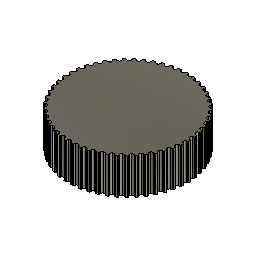
gear_53z (Autodesk Fusion 360 design; units mm, degrees)
Autodesk Fusion 360 part; units mm, degrees
sketch "Sketch1" plane through (0, 0, 0) normal (0, 0, 1) x (1, 0, 0) in component "gt2 pulley"
  circle A0 centre (0, 0) radius 16.8704 construction
  circle A1 centre (0, 0) radius 15.8664 construction
  line L0 (0, 0) -> (0, 16.8704) construction
  line L1 (0, 0) -> (0.9994, 16.8408) construction
  line L2 (0, 0) -> (1.4069, 16.8117) construction
  circle A2 centre (0, 0) radius 16.6164 construction
  arc A3 (0.389, 16.4769) -> (0.4579, 16.1856) centre (1.3857, 16.5585) ccw
  circle A4 centre (0, 0) radius 16.4664 construction
  arc A5 (0.2417, 16.6147) -> (0, 16.6164) centre (0, 0) ccw
  arc A6 (0.389, 16.4769) -> (0.2417, 16.6147) centre (0.2395, 16.4647) ccw
  arc A7 (0.4579, 16.1856) -> (0.9399, 15.8386) centre (0.9728, 16.3926) ccw
  arc A8 (0, 16.6164) -> (-0.2417, 16.6147) centre (0, 0) ccw
  arc A9 (-0.2417, 16.6147) -> (-0.389, 16.4769) centre (-0.2395, 16.4647) ccw
  arc A10 (-0.4579, 16.1856) -> (-0.389, 16.4769) centre (-1.3857, 16.5585) ccw
  arc A11 (-0.9399, 15.8386) -> (-0.4579, 16.1856) centre (-0.9728, 16.3926) ccw
  arc A12 (0.9399, 15.8386) -> (-0.9399, 15.8386) centre (0, 0) ccw
  point P0 (1.3857, 16.5585)
  point P1 (0, 16.6164)
  dimension "d18" = 33.7408
  dimension "d19" = 3.396
  dimension "d22" = 1.004
  dimension "d24" = 0.75
  dimension "d26" = 1
  dimension "d27" = 0.15
  dimension "d28" = 0.15
  dimension "d47" = 0.555
  dimension "d52" = 3.812
  constraint coincident A0.centre A1.centre
  constraint coincident A0 L0.end
  constraint vertical L0
  constraint coincident A0 L1.end
  constraint coincident A0 L2.end
  constraint concentric A1 A2
  constraint coincident A1 A7.end
  constraint coincident L1 A7.end
  constraint coincident A2 P0
  constraint coincident L2 P0
  constraint coincident P0 A3.centre
  constraint coincident A2 P1
  constraint coincident L0 P1
  constraint concentric A2 A4
  constraint coincident P1 A5.end
  constraint coincident A4 A6.centre
  constraint coincident A3.start A6.start
  constraint tangent A3 A6
  constraint tangent A3 A7
  constraint symmetric L0 A7.end A11.start
  constraint symmetric L0 A3.start A9.end
  constraint symmetric L0 A3.end A10.start
  constraint symmetric L0 A3 A10
  constraint symmetric L0 A5.start A8.end
  constraint symmetric L0 P1 A5.end
  constraint symmetric L0 A5 A8
  constraint symmetric L0 A6 A9
  constraint symmetric L0 A7 A11
  constraint coincident A1 A11.start
  constraint tangent A1 A7
  constraint coincident L1 A7.centre
  measures "d18" diameter of A0
  measures "d19" angle of L0 L1
  measures "d22" distance of A0 A1
  measures "d24" distance of A1 A2
  measures "d26" radius of A3
  measures "d27" distance of A2 A4
  measures "d28" radius of A6
  measures "d47" radius of A7
extrude "Extrude1" add sketch "Sketch1" along normal blind 10 makes body 1
pattern_circular "C-Pattern1" count 53 over 360 about axis through (0, 0, 1.75) along (0, 0, 1) of bodies 1 makes body 2 at (-1.9803, 15.7424, 6.6667) makes body 3 at (-3.0121, 15.5779, 3.3333) makes body 4 at (-4.8334, 15.1123, 3.3333) makes body 5 at (-7.3379, 14.0677, 6.6667) makes body 6 at (-8.2478, 13.5542, 3.3333) makes body 7 at (-10.9009, 11.5289, 6.6667) makes body 8 at (-11.2008, 11.2377, 3.3333) makes body 9 at (-12.9519, 9.1647, 6.6667) makes body 10 at (-13.9449, 7.5685, 6.6667) makes body 11 at (-14.4128, 6.6343, 3.3333) makes body 12 at (-15.3325, 4.0813, 6.6667) makes body 13 at (-15.5679, 3.0634, 3.3333) makes body 14 at (-15.8622, 0.3657, 6.6667) makes body 15 at (-15.7941, -1.5129, 6.6667) makes body 16 at (-15.6603, -2.5491, 3.3333) makes body 17 at (-15.2489, -4.3834, 3.3333) makes body 18 at (-14.2789, -6.9178, 6.6667) makes body 19 at (-13.012, -9.0792, 6.6667) makes body 20 at (-12.7683, -9.4188, 3.3333) makes body 21 at (-11.5647, -10.8628, 3.3333) makes body 22 at (-9.5445, -12.6746, 6.6667) makes body 23 at (-7.9784, -13.7145, 6.6667) makes body 24 at (-6.3004, -14.5619, 6.6667) makes body 25 at (-5.3283, -14.945, 3.3333) makes body 26 at (-2.0839, -15.729, 6.6667) makes body 27 at (-0.8356, -15.8444, 6.6667) makes body 28 at (1.0442, -15.832, 6.6667) makes body 29 at (2.0839, -15.729, 3.3333) makes body 30 at (4.7337, -15.1438, 6.6667) makes body 31 at (5.7201, -14.7994, 3.3333) makes body 32 at (8.1584, -13.6082, 6.6667) makes body 33 at (10.1987, -12.1544, 6.6667) makes body 34 at (10.5154, -11.8815, 3.3333) makes body 35 at (12.7683, -9.4188, 6.6667) makes body 36 at (13.012, -9.0792, 3.3333) makes body 37 at (13.9945, -7.4765, 3.3333) makes body 38 at (15.2489, -4.3834, 6.6667) makes body 39 at (15.6603, -2.5491, 6.6667) makes body 40 at (15.8127, -1.3048, 6.6667) makes body 41 at (15.856, 0.5746, 6.6667) makes body 42 at (15.7838, 1.6169, 3.3333) makes body 43 at (15.4818, 3.4724, 3.3333) makes body 44 at (14.6637, 6.0597, 6.6667) makes body 45 at (14.2331, 7.0117, 3.3333) makes body 46 at (12.8301, 9.3345, 6.6667) makes body 47 at (12.1879, 10.1587, 3.3333) makes body 48 at (10.9009, 11.5289, 3.3333) makes body 49 at (8.2478, 13.5542, 6.6667) makes body 50 at (7.1519, 14.1631, 6.6667) makes body 51 at (5.4266, 14.9096, 6.6667) makes body 52 at (4.4336, 15.2344, 3.3333) makes body 53 at (1.7728, 15.7671, 6.6667)
sketch "Sketch2" plane through (0, 0, 10) normal (0, 0, 1) x (-1, 0, 0)
  arc A0 (-11.0512, -12.2275) -> (-11.0295, -12.428) centre (-10.93, -12.3158) ccw
  arc A1 (-11.0295, -12.428) -> (-10.6634, -12.7436) centre (0, 0) ccw
  arc A2 (-10.6634, -12.7436) -> (-10.4618, -12.7354) centre (-10.567, -12.6286) ccw
  arc A3 (-10.2195, -12.5597) -> (-10.4618, -12.7354) centre (-9.7601, -13.4479) ccw
  arc A4 (-9.6277, -12.6115) -> (-10.2195, -12.5597) centre (-9.9645, -13.0526) ccw
  arc A5 (-11.0518, -11.3843) -> (-9.6277, -12.6115) centre (0, 0) ccw
  arc A6 (-10.9131, -11.9619) -> (-11.0518, -11.3843) centre (-11.4384, -11.7825) ccw
  arc A7 (-11.0512, -12.2275) -> (-10.9131, -11.9619) centre (-11.8595, -11.6387) ccw
  circle A8 centre (0, 0) radius 15.8664
  constraint concentric A1 A8
extrude "Extrude2" add sketch "Sketch2" against normal blind 10 contours A5 A8 bodies 1 2 3 4 5 6 7 8 9 10 11 12 13 14 15 16 17 18 19 20 21 22 23 24 25 26 27 28 29 30 31 32 33 34 35 36 37 38 39 40 41 42 43 44 45 46 47 48 49 50 51 52 53
extrude "Extrude4" [suppressed] in component "gt2 pulley"
pattern_circular "C-Pattern7" [suppressed] in component "gt2 pulley"
extrude "Extrude3" [suppressed] in component "gt2 pulley"
pattern_circular "C-Pattern6" [suppressed] in component "gt2 pulley"
extrude "Extrude2'" [suppressed] in component "gt2 pulley"
pattern_circular "C-Pattern5" [suppressed] in component "gt2 pulley"
extrude "Extrude1'" [suppressed] in component "gt2 pulley"
pattern_circular "C-Pattern4" [suppressed] in component "gt2 pulley"
pattern_circular "C-Pattern3" [suppressed] in component "gt2 pulley"
pattern_circular "C-Pattern2" [suppressed] in component "gt2 pulley"
pattern_circular "C-Pattern1'" [suppressed] in component "gt2 pulley"
copy_body "Body->Comp1" [suppressed] in component "Component"
copy_body "Body->Comp2" [suppressed] in component "Component'"
copy_body "Body->Comp3" [suppressed] in component "Component''"
copy_body "Body->Comp4" [suppressed] in component "Component'''"
copy_body "Body->Comp5" [suppressed] in component "Component''''"
copy_body "Body->Comp6" [suppressed] in component "Component'''''"
copy_body "Body->Comp7" [suppressed] in component "Component''''''"
copy_body "Body->Comp8" [suppressed] in component "Component'''''''"
copy_body "Body->Comp9" [suppressed] in component "Component''''''''"
copy_body "Body->Comp10" [suppressed] in component "Component'''''''''"
copy_body "Body->Comp11" [suppressed] in component "Component''''''''''"
copy_body "Body->Comp12" [suppressed] in component "Component'''''''''''"
copy_body "Body->Comp13" [suppressed] in component "Component''''''''''''"
copy_body "Body->Comp14" [suppressed] in component "Component'''''''''''''"
copy_body "Body->Comp15" [suppressed] in component "Component''''''''''''''"
copy_body "Body->Comp16" [suppressed] in component "Component'''''''''''''''"
copy_body "Body->Comp17" [suppressed] in component "Component''''''''''''''''"
copy_body "Body->Comp18" [suppressed] in component "Component'''''''''''''''''"
copy_body "Body->Comp19" [suppressed] in component "Component''''''''''''''''''"
copy_body "Body->Comp20" [suppressed] in component "Component'''''''''''''''''''"
component "gt2 pulley" placed x (1, 0, 0) y (0, 1, 0) z (0, 0, 1) at (0, 0, 0)
equation "NumTeeth = 53" comment "min 20"
equation "ToothPitch = 2 mm"
equation "PullyDia = NumTeeth * ToothPitch / PI"
equation "ToothAng = ( ( 360 / NumTeeth ) * 1 deg )"
equation "TransOffsetAngle = ToothAng * 0.2"
equation "Sholulder_Radius = 0.15 mm"
equation "Root_Radius = 0.555 mm"
equation "TransRadius = 1 mm"
equation "ToolHeight = 0.75 mm"
equation "PLD = 0.254 mm"
equation "d18 = PullyDia"
equation "d19 = ToothAng / 2"
equation "d22 = PLD + ToolHeight"
equation "d24 = ToolHeight"
equation "d26 = TransRadius"
equation "d27 = Sholulder_Radius"
equation "d31 = NumTeeth"
equation "d33 = NumTeeth"
equation "d35 = NumTeeth"
equation "d37 = NumTeeth"
equation "d41 = NumTeeth"
equation "d45 = NumTeeth"
equation "d47 = Root_Radius"
equation "d50 = NumTeeth"
